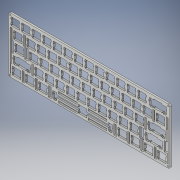
# Autodesk Inventor part: TopPlate
Saved by Autodesk Inventor 2019 (Build 230136000, 136)
## iProperties
Created: 2019-01-24
Part Number: TopPlate
Material: Generic
Document SubType Name: Modeling
Designer: Andrew
Density: 1 g/cm^3
Appearance: Default
Author: Andrew
Autodesk Inventor part; units mm, degrees
(part 1 of 2)
ref_plane "YZ Plane" through (0, 0, 0) normal (1, 0, 0) x (0, 1, 0)
ref_plane "XZ Plane" through (0, 0, 0) normal (0, 1, 0) x (-1, 0, 0)
ref_plane "XY Plane" through (0, 0, 0) normal (0, 0, 1) x (1, 0, 0)
sketch "Sketch1" plane through (0, 0, 0) normal (0, 0, 1) x (1, 0, 0)
  line L0 (290.7004, 97.1993) -> (290.7004, 3)
  arc A0 (287.7004, 0) -> (290.7004, 3) centre (287.7004, 3) ccw
  arc A1 (290.7004, 97.1993) -> (287.7004, 100.1993) centre (287.7004, 97.1993) ccw
  line L1 (126.4424, 18.9995) -> (126.4424, 17.999)
  line L2 (126.4424, 17.999) -> (125.6434, 17.999)
  line L3 (125.6434, 17.999) -> (125.6434, 14.299)
  line L4 (125.6434, 14.299) -> (86.8185, 14.299)
  line L5 (86.8185, 14.299) -> (86.8185, 17.5291)
  line L6 (86.8185, 17.5291) -> (80.0688, 17.5291)
  line L7 (80.0688, 17.5291) -> (80.0688, 14.299)
  line L8 (80.0688, 14.299) -> (79.2433, 14.299)
  line L9 (79.2433, 14.299) -> (79.2433, 11.4989)
  line L10 (79.2433, 11.4989) -> (80.0688, 11.4989)
  line L11 (80.0688, 11.4989) -> (80.0688, 5.2301)
  line L12 (80.0688, 5.2301) -> (81.7924, 5.2301)
  line L13 (81.7924, 5.2301) -> (81.7924, 4.0299)
  line L14 (81.7924, 4.0299) -> (85.093, 4.0299)
  line L15 (85.093, 4.0299) -> (85.093, 5.2301)
  line L16 (85.093, 5.2301) -> (86.8185, 5.2301)
  line L17 (86.8185, 5.2301) -> (86.8185, 9.7005)
  line L18 (86.8185, 9.7005) -> (125.6434, 9.7005)
  line L19 (125.6434, 9.7005) -> (125.6434, 5.9991)
  line L20 (125.6434, 5.9991) -> (126.4424, 5.9991)
  line L21 (126.4424, 5.9991) -> (126.4424, 5)
  line L22 (126.4424, 5) -> (140.4434, 5)
  line L23 (140.4434, 5) -> (140.4434, 5.9991)
  line L24 (140.4434, 5.9991) -> (141.2424, 5.9991)
  line L25 (141.2424, 5.9991) -> (141.2424, 9.7005)
  line L26 (141.2424, 9.7005) -> (180.0694, 9.7005)
  line L27 (180.0694, 9.7005) -> (180.0694, 5.2301)
  line L28 (180.0694, 5.2301) -> (181.7924, 5.2301)
  line L29 (181.7924, 5.2301) -> (181.7924, 4.0299)
  line L30 (181.7924, 4.0299) -> (185.0934, 4.0299)
  line L31 (185.0934, 4.0299) -> (185.0934, 5.2301)
  line L32 (185.0934, 5.2301) -> (186.8184, 5.2301)
  line L33 (186.8184, 5.2301) -> (186.8184, 11.4989)
  line L34 (186.8184, 11.4989) -> (187.6424, 11.4989)
  line L35 (187.6424, 11.4989) -> (187.6424, 14.299)
  line L36 (187.6424, 14.299) -> (186.8184, 14.299)
  line L37 (186.8184, 14.299) -> (186.8184, 17.5291)
  line L38 (186.8184, 17.5291) -> (180.0694, 17.5291)
  line L39 (180.0694, 17.5291) -> (180.0694, 14.299)
  line L40 (180.0694, 14.299) -> (141.2424, 14.299)
  line L41 (141.2424, 14.299) -> (141.2424, 17.999)
  line L42 (141.2424, 17.999) -> (140.4434, 17.999)
  line L43 (140.4434, 17.999) -> (140.4434, 18.9995)
  line L44 (140.4434, 18.9995) -> (126.4424, 18.9995)
  line L45 (7.3813, 18.9995) -> (7.3813, 17.999)
  line L46 (7.3813, 17.999) -> (6.5806, 17.999)
  line L47 (6.5806, 17.999) -> (6.5806, 14.8998)
  line L48 (6.5806, 14.8998) -> (7.3813, 14.8998)
  line L49 (7.3813, 14.8998) -> (7.3813, 9.0997)
  line L50 (7.3813, 9.0997) -> (6.5806, 9.0997)
  line L51 (6.5806, 9.0997) -> (6.5806, 5.9991)
  line L52 (6.5806, 5.9991) -> (7.3813, 5.9991)
  line L53 (7.3813, 5.9991) -> (7.3813, 5)
  line L54 (7.3813, 5) -> (21.3808, 5)
  line L55 (21.3808, 5) -> (21.3808, 5.9991)
  line L56 (21.3808, 5.9991) -> (22.1814, 5.9991)
  line L57 (22.1814, 5.9991) -> (22.1814, 9.0997)
  line L58 (22.1814, 9.0997) -> (21.3808, 9.0997)
  line L59 (21.3808, 9.0997) -> (21.3808, 14.8998)
  line L60 (21.3808, 14.8998) -> (22.1814, 14.8998)
  line L61 (22.1814, 14.8998) -> (22.1814, 17.999)
  line L62 (22.1814, 17.999) -> (21.3808, 17.999)
  line L63 (21.3808, 17.999) -> (21.3808, 18.9995)
  line L64 (21.3808, 18.9995) -> (7.3813, 18.9995)
  line L65 (31.1938, 18.9995) -> (31.1938, 17.999)
  line L66 (31.1938, 17.999) -> (30.3932, 17.999)
  line L67 (30.3932, 17.999) -> (30.3932, 14.8998)
  line L68 (30.3932, 14.8998) -> (31.1938, 14.8998)
  line L69 (31.1938, 14.8998) -> (31.1938, 9.0997)
  line L70 (31.1938, 9.0997) -> (30.3932, 9.0997)
  line L71 (30.3932, 9.0997) -> (30.3932, 5.9991)
  line L72 (30.3932, 5.9991) -> (31.1938, 5.9991)
  line L73 (31.1938, 5.9991) -> (31.1938, 5)
  line L74 (31.1938, 5) -> (45.1932, 5)
  line L75 (45.1932, 5) -> (45.1932, 5.9991)
  line L76 (45.1932, 5.9991) -> (45.9926, 5.9991)
  line L77 (45.9926, 5.9991) -> (45.9926, 9.0997)
  line L78 (45.9926, 9.0997) -> (45.1932, 9.0997)
  line L79 (45.1932, 9.0997) -> (45.1932, 14.8998)
  line L80 (45.1932, 14.8998) -> (45.9926, 14.8998)
  line L81 (45.9926, 14.8998) -> (45.9926, 17.999)
  line L82 (45.9926, 17.999) -> (45.1932, 17.999)
  line L83 (45.1932, 17.999) -> (45.1932, 18.9995)
  line L84 (45.1932, 18.9995) -> (31.1938, 18.9995)
  line L85 (55.0064, 18.9995) -> (55.0064, 17.999)
  line L86 (55.0064, 17.999) -> (54.2056, 17.999)
  line L87 (54.2056, 17.999) -> (54.2056, 14.8998)
  line L88 (54.2056, 14.8998) -> (55.0064, 14.8998)
  line L89 (55.0064, 14.8998) -> (55.0064, 9.0997)
  line L90 (55.0064, 9.0997) -> (54.2056, 9.0997)
  line L91 (54.2056, 9.0997) -> (54.2056, 5.9991)
  line L92 (54.2056, 5.9991) -> (55.0064, 5.9991)
  line L93 (55.0064, 5.9991) -> (55.0064, 5)
  line L94 (55.0064, 5) -> (69.0057, 5)
  line L95 (3, 0) -> (287.7004, 0)
  arc A2 (0, 3) -> (3, 0) centre (3, 3) ccw
  line L96 (69.0057, 5) -> (69.0057, 5.9991)
  line L97 (69.0057, 5.9991) -> (69.8065, 5.9991)
  line L98 (69.8065, 5.9991) -> (69.8065, 9.0997)
  line L99 (69.8065, 9.0997) -> (69.0057, 9.0997)
  line L100 (69.0057, 9.0997) -> (69.0057, 14.8998)
  line L101 (69.0057, 14.8998) -> (69.8065, 14.8998)
  line L102 (69.8065, 14.8998) -> (69.8065, 17.999)
  line L103 (69.8065, 17.999) -> (69.0057, 17.999)
  line L104 (69.0057, 17.999) -> (69.0057, 18.9995)
  line L105 (69.0057, 18.9995) -> (55.0064, 18.9995)
  line L106 (197.8814, 18.9995) -> (197.8814, 17.999)
  line L107 (197.8814, 17.999) -> (197.0804, 17.999)
  line L108 (197.0804, 17.999) -> (197.0804, 14.8998)
  line L109 (197.0804, 14.8998) -> (197.8814, 14.8998)
  line L110 (197.8814, 14.8998) -> (197.8814, 9.0997)
  line L111 (197.8814, 9.0997) -> (197.0804, 9.0997)
  line L112 (197.0804, 9.0997) -> (197.0804, 5.9991)
  line L113 (197.0804, 5.9991) -> (197.8814, 5.9991)
  line L114 (197.8814, 5.9991) -> (197.8814, 5)
  line L115 (197.8814, 5) -> (211.8804, 5)
  line L116 (211.8804, 5) -> (211.8804, 5.9991)
  line L117 (211.8804, 5.9991) -> (212.6814, 5.9991)
  line L118 (212.6814, 5.9991) -> (212.6814, 9.0997)
  line L119 (212.6814, 9.0997) -> (211.8804, 9.0997)
  line L120 (211.8804, 9.0997) -> (211.8804, 14.8998)
  line L121 (211.8804, 14.8998) -> (212.6814, 14.8998)
  line L122 (212.6814, 14.8998) -> (212.6814, 17.999)
  line L123 (212.6814, 17.999) -> (211.8804, 17.999)
  line L124 (211.8804, 17.999) -> (211.8804, 18.9995)
  line L125 (211.8804, 18.9995) -> (197.8814, 18.9995)
  line L126 (221.6934, 18.9995) -> (221.6934, 17.999)
  line L127 (221.6934, 17.999) -> (220.8934, 17.999)
  line L128 (220.8934, 17.999) -> (220.8934, 14.8998)
  line L129 (220.8934, 14.8998) -> (221.6934, 14.8998)
  line L130 (221.6934, 14.8998) -> (221.6934, 9.0997)
  line L131 (221.6934, 9.0997) -> (220.8934, 9.0997)
  line L132 (220.8934, 9.0997) -> (220.8934, 5.9991)
  line L133 (220.8934, 5.9991) -> (221.6934, 5.9991)
  line L134 (221.6934, 5.9991) -> (221.6934, 5)
  line L135 (221.6934, 5) -> (235.6934, 5)
  line L136 (235.6934, 5) -> (235.6934, 5.9991)
  line L137 (235.6934, 5.9991) -> (236.4924, 5.9991)
  line L138 (236.4924, 5.9991) -> (236.4924, 9.0997)
  line L139 (236.4924, 9.0997) -> (235.6934, 9.0997)
  line L140 (235.6934, 9.0997) -> (235.6934, 14.8998)
  line L141 (235.6934, 14.8998) -> (236.4924, 14.8998)
  line L142 (236.4924, 14.8998) -> (236.4924, 17.999)
  line L143 (236.4924, 17.999) -> (235.6934, 17.999)
  line L144 (235.6934, 17.999) -> (235.6934, 18.9995)
  line L145 (235.6934, 18.9995) -> (221.6934, 18.9995)
  line L146 (245.5064, 18.9995) -> (245.5064, 17.999)
  line L147 (245.5064, 17.999) -> (244.7054, 17.999)
  line L148 (244.7054, 17.999) -> (244.7054, 14.8998)
  line L149 (244.7054, 14.8998) -> (245.5064, 14.8998)
  line L150 (245.5064, 14.8998) -> (245.5064, 9.0997)
  line L151 (245.5064, 9.0997) -> (244.7054, 9.0997)
  line L152 (244.7054, 9.0997) -> (244.7054, 5.9991)
  line L153 (244.7054, 5.9991) -> (245.5064, 5.9991)
  line L154 (245.5064, 5.9991) -> (245.5064, 5)
  line L155 (245.5064, 5) -> (259.5054, 5)
  line L156 (259.5054, 5) -> (259.5054, 5.9991)
  line L157 (259.5054, 5.9991) -> (260.3064, 5.9991)
  line L158 (260.3064, 5.9991) -> (260.3064, 9.0997)
  line L159 (260.3064, 9.0997) -> (259.5054, 9.0997)
  line L160 (259.5054, 9.0997) -> (259.5054, 14.8998)
  line L161 (259.5054, 14.8998) -> (260.3064, 14.8998)
  line L162 (260.3064, 14.8998) -> (260.3064, 17.999)
  line L163 (260.3064, 17.999) -> (259.5054, 17.999)
  line L164 (259.5054, 17.999) -> (259.5054, 18.9995)
  line L165 (259.5054, 18.9995) -> (245.5064, 18.9995)
  line L166 (269.3184, 18.9995) -> (269.3184, 17.999)
  line L167 (269.3184, 17.999) -> (268.5184, 17.999)
  line L168 (268.5184, 17.999) -> (268.5184, 14.8998)
  line L169 (268.5184, 14.8998) -> (269.3184, 14.8998)
  line L170 (269.3184, 14.8998) -> (269.3184, 9.0997)
  line L171 (269.3184, 9.0997) -> (268.5184, 9.0997)
  line L172 (268.5184, 9.0997) -> (268.5184, 5.9991)
  line L173 (268.5184, 5.9991) -> (269.3184, 5.9991)
  line L174 (269.3184, 5.9991) -> (269.3184, 5)
  line L175 (269.3184, 5) -> (283.3184, 5)
  line L176 (283.3184, 5) -> (283.3184, 5.9991)
  line L177 (283.3184, 5.9991) -> (284.1174, 5.9991)
  line L178 (284.1174, 5.9991) -> (284.1174, 9.0997)
  line L179 (284.1174, 9.0997) -> (283.3184, 9.0997)
  line L180 (283.3184, 9.0997) -> (283.3184, 14.8998)
  line L181 (283.3184, 14.8998) -> (284.1174, 14.8998)
  line L182 (284.1174, 14.8998) -> (284.1174, 17.999)
  line L183 (284.1174, 17.999) -> (283.3184, 17.999)
  line L184 (283.3184, 17.999) -> (283.3184, 18.9995)
  line L185 (283.3184, 18.9995) -> (269.3184, 18.9995)
  line L186 (16.9063, 38.0493) -> (16.9063, 37.049)
  line L187 (16.9063, 37.049) -> (16.1057, 37.049)
  line L188 (16.1057, 36.5791) -> (8.6312, 36.5791)
  line L189 (8.6312, 36.5791) -> (8.6312, 33.349)
  line L190 (8.6312, 33.349) -> (7.8057, 33.349)
  line L191 (7.8057, 33.349) -> (7.8057, 30.5488)
  line L192 (7.8057, 30.5488) -> (8.6312, 30.5488)
  line L193 (8.6312, 30.5488) -> (8.6312, 24.2787)
  line L194 (8.6312, 24.2787) -> (10.3564, 24.2787)
  line L195 (10.3564, 24.2787) -> (10.3564, 23.0798)
  line L196 (10.3564, 23.0798) -> (13.6555, 23.0798)
  line L197 (13.6555, 23.0798) -> (13.6555, 24.2787)
  line L198 (13.6555, 24.2787) -> (15.3808, 24.2787)
  line L199 (15.3808, 25.049) -> (16.9063, 25.049)
  line L200 (16.9063, 25.049) -> (16.9063, 24.05)
  line L201 (16.9063, 24.05) -> (30.9058, 24.05)
  line L202 (30.9058, 24.05) -> (30.9058, 25.049)
  line L203 (30.9058, 25.049) -> (32.4313, 25.049)
  line L204 (32.4313, 24.2787) -> (34.1566, 24.2787)
  line L205 (34.1566, 24.2787) -> (34.1566, 23.0798)
  line L206 (34.1566, 23.0798) -> (37.4556, 23.0798)
  line L207 (37.4556, 23.0798) -> (37.4556, 24.2787)
  line L208 (37.4556, 24.2787) -> (39.1808, 24.2787)
  line L209 (39.1808, 24.2787) -> (39.1808, 30.5488)
  line L210 (39.1808, 30.5488) -> (40.0063, 30.5488)
  line L211 (40.0063, 30.5488) -> (40.0063, 33.349)
  line L212 (40.0063, 33.349) -> (39.1808, 33.349)
  line L213 (39.1808, 33.349) -> (39.1808, 36.5791)
  line L214 (39.1808, 36.5791) -> (31.7064, 36.5791)
  line L215 (31.7064, 37.049) -> (30.9058, 37.049)
  line L216 (30.9058, 37.049) -> (30.9058, 38.0493)
  line L217 (30.9058, 38.0493) -> (16.9063, 38.0493)
  line L218 (255.0304, 38.0493) -> (255.0304, 37.049)
  line L219 (255.0304, 37.049) -> (254.2304, 37.049)
  line L220 (254.2304, 36.5791) -> (246.7564, 36.5791)
  line L221 (246.7564, 36.5791) -> (246.7564, 33.349)
  line L222 (246.7564, 33.349) -> (245.9304, 33.349)
  line L223 (245.9304, 33.349) -> (245.9304, 30.5488)
  line L224 (245.9304, 30.5488) -> (246.7564, 30.5488)
  line L225 (246.7564, 30.5488) -> (246.7564, 24.2787)
  line L226 (246.7564, 24.2787) -> (248.4814, 24.2787)
  line L227 (248.4814, 24.2787) -> (248.4814, 23.0798)
  line L228 (248.4814, 23.0798) -> (251.7804, 23.0798)
  line L229 (251.7804, 23.0798) -> (251.7804, 24.2787)
  line L230 (251.7804, 24.2787) -> (253.5064, 24.2787)
  line L231 (253.5064, 25.049) -> (255.0304, 25.049)
  line L232 (255.0304, 25.049) -> (255.0304, 24.05)
  line L233 (255.0304, 24.05) -> (269.0304, 24.05)
  line L234 (269.0304, 24.05) -> (269.0304, 25.049)
  line L235 (269.0304, 25.049) -> (270.5564, 25.049)
  line L236 (270.5564, 24.2787) -> (272.2814, 24.2787)
  line L237 (272.2814, 24.2787) -> (272.2814, 23.0798)
  line L238 (272.2814, 23.0798) -> (275.5804, 23.0798)
  line L239 (275.5804, 23.0798) -> (275.5804, 24.2787)
  line L240 (275.5804, 24.2787) -> (277.3054, 24.2787)
  line L241 (277.3054, 24.2787) -> (277.3054, 30.5488)
  line L242 (277.3054, 30.5488) -> (278.1314, 30.5488)
  line L243 (278.1314, 30.5488) -> (278.1314, 33.349)
  line L244 (278.1314, 33.349) -> (277.3054, 33.349)
  line L245 (277.3054, 33.349) -> (277.3054, 36.5791)
  line L246 (277.3054, 36.5791) -> (269.8314, 36.5791)
  line L247 (269.8314, 37.049) -> (269.0304, 37.049)
  line L248 (269.0304, 37.049) -> (269.0304, 38.0493)
  line L249 (269.0304, 38.0493) -> (255.0304, 38.0493)
  line L250 (47.8626, 38.0493) -> (47.8626, 37.049)
  line L251 (47.8626, 37.049) -> (47.0618, 37.049)
  line L252 (47.0618, 37.049) -> (47.0618, 33.9498)
  line L253 (47.0618, 33.9498) -> (47.8626, 33.9498)
  line L254 (47.8626, 33.9498) -> (47.8626, 28.1496)
  line L255 (47.8626, 28.1496) -> (47.0618, 28.1496)
  line L256 (47.0618, 28.1496) -> (47.0618, 25.049)
  line L257 (47.0618, 25.049) -> (47.8626, 25.049)
  line L258 (47.8626, 25.049) -> (47.8626, 24.05)
  line L259 (47.8626, 24.05) -> (61.8619, 24.05)
  line L260 (61.8619, 24.05) -> (61.8619, 25.049)
  line L261 (61.8619, 25.049) -> (62.6627, 25.049)
  line L262 (62.6627, 25.049) -> (62.6627, 28.1496)
  line L263 (62.6627, 28.1496) -> (61.8619, 28.1496)
  line L264 (61.8619, 28.1496) -> (61.8619, 33.9498)
  line L265 (61.8619, 33.9498) -> (62.6627, 33.9498)
  line L266 (62.6627, 33.9498) -> (62.6627, 37.049)
  line L267 (62.6627, 37.049) -> (61.8619, 37.049)
  line L268 (61.8619, 37.049) -> (61.8619, 38.0493)
  line L269 (61.8619, 38.0493) -> (47.8626, 38.0493)
  line L270 (66.9126, 38.0493) -> (66.9126, 37.049)
  line L271 (66.9126, 37.049) -> (66.1118, 37.049)
  line L272 (66.1118, 37.049) -> (66.1118, 33.9498)
  line L273 (66.1118, 33.9498) -> (66.9126, 33.9498)
  line L274 (66.9126, 33.9498) -> (66.9126, 28.1496)
  line L275 (66.9126, 28.1496) -> (66.1118, 28.1496)
  line L276 (66.1118, 28.1496) -> (66.1118, 25.049)
  line L277 (66.1118, 25.049) -> (66.9126, 25.049)
  line L278 (66.9126, 25.049) -> (66.9126, 24.05)
  line L279 (66.9126, 24.05) -> (80.9119, 24.05)
  line L280 (80.9119, 24.05) -> (80.9119, 25.049)
  line L281 (80.9119, 25.049) -> (81.7127, 25.049)
  line L282 (81.7127, 25.049) -> (81.7127, 28.1496)
  line L283 (81.7127, 28.1496) -> (80.9119, 28.1496)
  line L284 (80.9119, 28.1496) -> (80.9119, 33.9498)
  line L285 (80.9119, 33.9498) -> (81.7127, 33.9498)
  line L286 (81.7127, 33.9498) -> (81.7127, 37.049)
  line L287 (81.7127, 37.049) -> (80.9119, 37.049)
  line L288 (80.9119, 37.049) -> (80.9119, 38.0493)
  line L289 (80.9119, 38.0493) -> (66.9126, 38.0493)
  line L290 (85.9626, 38.0493) -> (85.9626, 37.049)
  line L291 (85.9626, 37.049) -> (85.1618, 37.049)
  line L292 (85.1618, 37.049) -> (85.1618, 33.9498)
  line L293 (85.1618, 33.9498) -> (85.9626, 33.9498)
  line L294 (85.9626, 33.9498) -> (85.9626, 28.1496)
  line L295 (85.9626, 28.1496) -> (85.1618, 28.1496)
  line L296 (85.1618, 28.1496) -> (85.1618, 25.049)
  line L297 (85.1618, 25.049) -> (85.9626, 25.049)
  line L298 (85.9626, 25.049) -> (85.9626, 24.05)
  line L299 (85.9626, 24.05) -> (99.9619, 24.05)
  line L300 (99.9619, 24.05) -> (99.9619, 25.049)
  line L301 (99.9619, 25.049) -> (100.7627, 25.049)
  line L302 (100.7627, 25.049) -> (100.7627, 28.1496)
  line L303 (100.7627, 28.1496) -> (99.9619, 28.1496)
  line L304 (99.9619, 28.1496) -> (99.9619, 33.9498)
  line L305 (99.9619, 33.9498) -> (100.7627, 33.9498)
  line L306 (100.7627, 33.9498) -> (100.7627, 37.049)
  line L307 (100.7627, 37.049) -> (99.9619, 37.049)
  line L308 (99.9619, 37.049) -> (99.9619, 38.0493)
  line L309 (99.9619, 38.0493) -> (85.9626, 38.0493)
  line L310 (105.0124, 38.0493) -> (105.0124, 37.049)
  line L311 (105.0124, 37.049) -> (104.2114, 37.049)
  line L312 (104.2114, 37.049) -> (104.2114, 33.9498)
  line L313 (104.2114, 33.9498) -> (105.0124, 33.9498)
  line L314 (105.0124, 33.9498) -> (105.0124, 28.1496)
  line L315 (105.0124, 28.1496) -> (104.2114, 28.1496)
  line L316 (104.2114, 28.1496) -> (104.2114, 25.049)
  line L317 (104.2114, 25.049) -> (105.0124, 25.049)
  line L318 (105.0124, 25.049) -> (105.0124, 24.05)
  line L319 (105.0124, 24.05) -> (119.0124, 24.05)
  line L320 (119.0124, 24.05) -> (119.0124, 25.049)
  line L321 (119.0124, 25.049) -> (119.8124, 25.049)
  line L322 (119.8124, 25.049) -> (119.8124, 28.1496)
  line L323 (119.8124, 28.1496) -> (119.0124, 28.1496)
  line L324 (119.0124, 28.1496) -> (119.0124, 33.9498)
  line L325 (119.0124, 33.9498) -> (119.8124, 33.9498)
  line L326 (119.8124, 33.9498) -> (119.8124, 37.049)
  line L327 (119.8124, 37.049) -> (119.0124, 37.049)
  line L328 (119.0124, 37.049) -> (119.0124, 38.0493)
  line L329 (119.0124, 38.0493) -> (105.0124, 38.0493)
  line L330 (124.0624, 38.0493) -> (124.0624, 37.049)
  line L331 (124.0624, 37.049) -> (123.2614, 37.049)
  line L332 (123.2614, 37.049) -> (123.2614, 33.9498)
  line L333 (123.2614, 33.9498) -> (124.0624, 33.9498)
  line L334 (124.0624, 33.9498) -> (124.0624, 28.1496)
  line L335 (124.0624, 28.1496) -> (123.2614, 28.1496)
  line L336 (123.2614, 28.1496) -> (123.2614, 25.049)
  line L337 (123.2614, 25.049) -> (124.0624, 25.049)
  line L338 (124.0624, 25.049) -> (124.0624, 24.05)
  line L339 (124.0624, 24.05) -> (138.0624, 24.05)
  line L340 (138.0624, 24.05) -> (138.0624, 25.049)
  line L341 (138.0624, 25.049) -> (138.8624, 25.049)
  line L342 (138.8624, 25.049) -> (138.8624, 28.1496)
  line L343 (138.8624, 28.1496) -> (138.0624, 28.1496)
  line L344 (138.0624, 28.1496) -> (138.0624, 33.9498)
  line L345 (138.0624, 33.9498) -> (138.8624, 33.9498)
  line L346 (138.8624, 33.9498) -> (138.8624, 37.049)
  line L347 (138.8624, 37.049) -> (138.0624, 37.049)
  line L348 (138.0624, 37.049) -> (138.0624, 38.0493)
  line L349 (138.0624, 38.0493) -> (124.0624, 38.0493)
  line L350 (143.1124, 38.0493) -> (143.1124, 37.049)
  line L351 (143.1124, 37.049) -> (142.3114, 37.049)
  line L352 (142.3114, 37.049) -> (142.3114, 33.9498)
  line L353 (142.3114, 33.9498) -> (143.1124, 33.9498)
  line L354 (143.1124, 33.9498) -> (143.1124, 28.1496)
  line L355 (143.1124, 28.1496) -> (142.3114, 28.1496)
  line L356 (142.3114, 28.1496) -> (142.3114, 25.049)
  line L357 (142.3114, 25.049) -> (143.1124, 25.049)
  line L358 (143.1124, 25.049) -> (143.1124, 24.05)
  line L359 (143.1124, 24.05) -> (157.1124, 24.05)
  line L360 (157.1124, 24.05) -> (157.1124, 25.049)
  line L361 (157.1124, 25.049) -> (157.9124, 25.049)
  line L362 (157.9124, 25.049) -> (157.9124, 28.1496)
  line L363 (157.9124, 28.1496) -> (157.1124, 28.1496)
  line L364 (157.1124, 28.1496) -> (157.1124, 33.9498)
  line L365 (157.1124, 33.9498) -> (157.9124, 33.9498)
  line L366 (157.9124, 33.9498) -> (157.9124, 37.049)
  line L367 (157.9124, 37.049) -> (157.1124, 37.049)
  line L368 (157.1124, 37.049) -> (157.1124, 38.0493)
  line L369 (157.1124, 38.0493) -> (143.1124, 38.0493)
  line L370 (162.1624, 38.0493) -> (162.1624, 37.049)
  line L371 (162.1624, 37.049) -> (161.3614, 37.049)
  line L372 (161.3614, 37.049) -> (161.3614, 33.9498)
  line L373 (161.3614, 33.9498) -> (162.1624, 33.9498)
  line L374 (162.1624, 33.9498) -> (162.1624, 28.1496)
  line L375 (162.1624, 28.1496) -> (161.3614, 28.1496)
  line L376 (161.3614, 28.1496) -> (161.3614, 25.049)
  line L377 (161.3614, 25.049) -> (162.1624, 25.049)
  line L378 (162.1624, 25.049) -> (162.1624, 24.05)
  line L379 (162.1624, 24.05) -> (176.1624, 24.05)
  line L380 (176.1624, 24.05) -> (176.1624, 25.049)
  line L381 (176.1624, 25.049) -> (176.9624, 25.049)
  line L382 (176.9624, 25.049) -> (176.9624, 28.1496)
  line L383 (176.9624, 28.1496) -> (176.1624, 28.1496)
  line L384 (176.1624, 28.1496) -> (176.1624, 33.9498)
  line L385 (176.1624, 33.9498) -> (176.9624, 33.9498)
  line L386 (176.9624, 33.9498) -> (176.9624, 37.049)
  line L387 (176.9624, 37.049) -> (176.1624, 37.049)
  line L388 (176.1624, 37.049) -> (176.1624, 38.0493)
  line L389 (176.1624, 38.0493) -> (162.1624, 38.0493)
  line L390 (181.2124, 38.0493) -> (181.2124, 37.049)
  line L391 (181.2124, 37.049) -> (180.4114, 37.049)
  line L392 (180.4114, 37.049) -> (180.4114, 33.9498)
  line L393 (180.4114, 33.9498) -> (181.2124, 33.9498)
  line L394 (181.2124, 33.9498) -> (181.2124, 28.1496)
  line L395 (181.2124, 28.1496) -> (180.4114, 28.1496)
  line L396 (180.4114, 28.1496) -> (180.4114, 25.049)
  line L397 (180.4114, 25.049) -> (181.2124, 25.049)
  line L398 (181.2124, 25.049) -> (181.2124, 24.05)
  line L399 (181.2124, 24.05) -> (195.2124, 24.05)
  line L400 (195.2124, 24.05) -> (195.2124, 25.049)
  line L401 (195.2124, 25.049) -> (196.0124, 25.049)
  line L402 (196.0124, 25.049) -> (196.0124, 28.1496)
  line L403 (196.0124, 28.1496) -> (195.2124, 28.1496)
  line L404 (195.2124, 28.1496) -> (195.2124, 33.9498)
  line L405 (195.2124, 33.9498) -> (196.0124, 33.9498)
  line L406 (196.0124, 33.9498) -> (196.0124, 37.049)
  line L407 (196.0124, 37.049) -> (195.2124, 37.049)
  line L408 (195.2124, 37.049) -> (195.2124, 38.0493)
  line L409 (195.2124, 38.0493) -> (181.2124, 38.0493)
  line L410 (200.2624, 38.0493) -> (200.2624, 37.049)
  line L411 (200.2624, 37.049) -> (199.4614, 37.049)
  line L412 (199.4614, 37.049) -> (199.4614, 33.9498)
  line L413 (199.4614, 33.9498) -> (200.2624, 33.9498)
  line L414 (200.2624, 33.9498) -> (200.2624, 28.1496)
  line L415 (200.2624, 28.1496) -> (199.4614, 28.1496)
  line L416 (199.4614, 28.1496) -> (199.4614, 25.049)
  line L417 (199.4614, 25.049) -> (200.2624, 25.049)
  line L418 (200.2624, 25.049) -> (200.2624, 24.05)
  line L419 (200.2624, 24.05) -> (214.2624, 24.05)
  line L420 (214.2624, 24.05) -> (214.2624, 25.049)
  line L421 (214.2624, 25.049) -> (215.0624, 25.049)
  line L422 (215.0624, 25.049) -> (215.0624, 28.1496)
  line L423 (215.0624, 28.1496) -> (214.2624, 28.1496)
  line L424 (214.2624, 28.1496) -> (214.2624, 33.9498)
  line L425 (214.2624, 33.9498) -> (215.0624, 33.9498)
  line L426 (215.0624, 33.9498) -> (215.0624, 37.049)
  line L427 (215.0624, 37.049) -> (214.2624, 37.049)
  line L428 (214.2624, 37.049) -> (214.2624, 38.0493)
  line L429 (214.2624, 38.0493) -> (200.2624, 38.0493)
  line L430 (219.3124, 38.0493) -> (219.3124, 37.049)
  line L431 (219.3124, 37.049) -> (218.5114, 37.049)
  line L432 (218.5114, 37.049) -> (218.5114, 33.9498)
  line L433 (218.5114, 33.9498) -> (219.3124, 33.9498)
  line L434 (219.3124, 33.9498) -> (219.3124, 28.1496)
  line L435 (219.3124, 28.1496) -> (218.5114, 28.1496)
  line L436 (218.5114, 28.1496) -> (218.5114, 25.049)
  line L437 (218.5114, 25.049) -> (219.3124, 25.049)
  line L438 (219.3124, 25.049) -> (219.3124, 24.05)
  line L439 (219.3124, 24.05) -> (233.3124, 24.05)
  line L440 (233.3124, 24.05) -> (233.3124, 25.049)
  line L441 (233.3124, 25.049) -> (234.1124, 25.049)
  line L442 (234.1124, 25.049) -> (234.1124, 28.1496)
  line L443 (234.1124, 28.1496) -> (233.3124, 28.1496)
  line L444 (233.3124, 28.1496) -> (233.3124, 33.9498)
  line L445 (233.3124, 33.9498) -> (234.1124, 33.9498)
  line L446 (234.1124, 33.9498) -> (234.1124, 37.049)
  line L447 (234.1124, 37.049) -> (233.3124, 37.049)
  line L448 (233.3124, 37.049) -> (233.3124, 38.0493)
  line L449 (233.3124, 38.0493) -> (219.3124, 38.0493)
  line L450 (259.7934, 57.0993) -> (259.7934, 56.0992)
  line L451 (259.7934, 56.0992) -> (258.9914, 56.0992)
  line L452 (258.9914, 56.0992) -> (258.9914, 55.6293)
  line L453 (258.9914, 55.6293) -> (251.5184, 55.6293)
  line L454 (251.5184, 55.6293) -> (251.5184, 52.3989)
  line L455 (251.5184, 52.3989) -> (250.6934, 52.3989)
  line L456 (250.6934, 52.3989) -> (250.6934, 49.5989)
  line L457 (250.6934, 49.5989) -> (251.5184, 49.5989)
  line L458 (251.5184, 49.5989) -> (251.5184, 43.33)
  line L459 (251.5184, 43.33) -> (253.2424, 43.33)
  line L460 (253.2424, 43.33) -> (253.2424, 42.1299)
  line L461 (253.2424, 42.1299) -> (256.5414, 42.1299)
  line L462 (256.5414, 42.1299) -> (256.5414, 43.33)
  line L463 (256.5414, 43.33) -> (258.2684, 43.33)
  line L464 (258.2684, 43.33) -> (258.2684, 44.0991)
  line L465 (258.2684, 44.0991) -> (259.7934, 44.0991)
  line L466 (259.7934, 44.0991) -> (259.7934, 43.1)
  line L467 (259.7934, 43.1) -> (273.7934, 43.1)
  line L468 (273.7934, 43.1) -> (273.7934, 44.0991)
  line L469 (273.7934, 44.0991) -> (275.3194, 44.0991)
  line L470 (275.3194, 44.0991) -> (275.3194, 43.33)
  line L471 (275.3194, 43.33) -> (277.0424, 43.33)
  line L472 (277.0424, 43.33) -> (277.0424, 42.1299)
  line L473 (277.0424, 42.1299) -> (280.3434, 42.1299)
  line L474 (280.3434, 42.1299) -> (280.3434, 43.33)
  line L475 (280.3434, 43.33) -> (282.0684, 43.33)
  line L476 (282.0684, 43.33) -> (282.0684, 49.5989)
  line L477 (282.0684, 49.5989) -> (282.8924, 49.5989)
  line L478 (282.8924, 49.5989) -> (282.8924, 52.3989)
  line L479 (282.8924, 52.3989) -> (282.0684, 52.3989)
  line L480 (282.0684, 52.3989) -> (282.0684, 55.6293)
  line L481 (282.0684, 55.6293) -> (274.5924, 55.6293)
  line L482 (274.5924, 55.6293) -> (274.5924, 56.0992)
  line L483 (274.5924, 56.0992) -> (273.7934, 56.0992)
  line L484 (273.7934, 56.0992) -> (273.7934, 57.0993)
  line L485 (273.7934, 57.0993) -> (259.7934, 57.0993)
  line L486 (12.1438, 57.0993) -> (12.1438, 56.0992)
  line L487 (12.1438, 56.0992) -> (11.3431, 56.0992)
  line L488 (11.3431, 56.0992) -> (11.3431, 52.9997)
  line L489 (11.3431, 52.9997) -> (12.1438, 52.9997)
  line L490 (12.1438, 52.9997) -> (12.1438, 47.1996)
  line L491 (12.1438, 47.1996) -> (11.3431, 47.1996)
  line L492 (11.3431, 47.1996) -> (11.3431, 44.0991)
  line L493 (11.3431, 44.0991) -> (12.1438, 44.0991)
  line L494 (12.1438, 44.0991) -> (12.1438, 43.1)
  line L495 (12.1438, 43.1) -> (26.1433, 43.1)
  line L496 (26.1433, 43.1) -> (26.1433, 44.0991)
  line L497 (26.1433, 44.0991) -> (26.9426, 44.0991)
  line L498 (26.9426, 44.0991) -> (26.9426, 47.1996)
  line L499 (26.9426, 47.1996) -> (26.1433, 47.1996)
  line L500 (26.1433, 47.1996) -> (26.1433, 52.9997)
  line L501 (26.1433, 52.9997) -> (26.9426, 52.9997)
  line L502 (26.9426, 52.9997) -> (26.9426, 56.0992)
  line L503 (26.9426, 56.0992) -> (26.1433, 56.0992)
  line L504 (26.1433, 56.0992) -> (26.1433, 57.0993)
  line L505 (26.1433, 57.0993) -> (12.1438, 57.0993)
  line L506 (38.3376, 57.0993) -> (38.3376, 56.0992)
  line L507 (38.3376, 56.0992) -> (37.5369, 56.0992)
  line L508 (37.5369, 56.0992) -> (37.5369, 52.9997)
  line L509 (37.5369, 52.9997) -> (38.3376, 52.9997)
  line L510 (38.3376, 52.9997) -> (38.3376, 47.1996)
  line L511 (38.3376, 47.1996) -> (37.5369, 47.1996)
  line L512 (37.5369, 47.1996) -> (37.5369, 44.0991)
  line L513 (37.5369, 44.0991) -> (38.3376, 44.0991)
  line L514 (38.3376, 44.0991) -> (38.3376, 43.1)
  line L515 (38.3376, 43.1) -> (52.3369, 43.1)
  line L516 (52.3369, 43.1) -> (52.3369, 44.0991)
  line L517 (52.3369, 44.0991) -> (53.1377, 44.0991)
  line L518 (53.1377, 44.0991) -> (53.1377, 47.1996)
  line L519 (53.1377, 47.1996) -> (52.3369, 47.1996)
  line L520 (52.3369, 47.1996) -> (52.3369, 52.9997)
  line L521 (52.3369, 52.9997) -> (53.1377, 52.9997)
  line L522 (53.1377, 52.9997) -> (53.1377, 56.0992)
  line L523 (53.1377, 56.0992) -> (52.3369, 56.0992)
  line L524 (52.3369, 56.0992) -> (52.3369, 57.0993)
  line L525 (52.3369, 57.0993) -> (38.3376, 57.0993)
  line L526 (57.3876, 57.0993) -> (57.3876, 56.0992)
  line L527 (57.3876, 56.0992) -> (56.5868, 56.0992)
  line L528 (56.5868, 56.0992) -> (56.5868, 52.9997)
  line L529 (56.5868, 52.9997) -> (57.3876, 52.9997)
  line L530 (57.3876, 52.9997) -> (57.3876, 47.1996)
  line L531 (57.3876, 47.1996) -> (56.5868, 47.1996)
  line L532 (56.5868, 47.1996) -> (56.5868, 44.0991)
  line L533 (56.5868, 44.0991) -> (57.3876, 44.0991)
  line L534 (57.3876, 44.0991) -> (57.3876, 43.1)
  line L535 (57.3876, 43.1) -> (71.3869, 43.1)
  line L536 (71.3869, 43.1) -> (71.3869, 44.0991)
  line L537 (71.3869, 44.0991) -> (72.1877, 44.0991)
  line L538 (72.1877, 44.0991) -> (72.1877, 47.1996)
  line L539 (72.1877, 47.1996) -> (71.3869, 47.1996)
  line L540 (71.3869, 47.1996) -> (71.3869, 52.9997)
  line L541 (71.3869, 52.9997) -> (72.1877, 52.9997)
  line L542 (72.1877, 52.9997) -> (72.1877, 56.0992)
  line L543 (72.1877, 56.0992) -> (71.3869, 56.0992)
  line L544 (71.3869, 56.0992) -> (71.3869, 57.0993)
  line L545 (71.3869, 57.0993) -> (57.3876, 57.0993)
  line L546 (76.4376, 57.0993) -> (76.4376, 56.0992)
  line L547 (76.4376, 56.0992) -> (75.6368, 56.0992)
  line L548 (75.6368, 56.0992) -> (75.6368, 52.9997)
  line L549 (75.6368, 52.9997) -> (76.4376, 52.9997)
  line L550 (76.4376, 52.9997) -> (76.4376, 47.1996)
  line L551 (76.4376, 47.1996) -> (75.6368, 47.1996)
  line L552 (75.6368, 47.1996) -> (75.6368, 44.0991)
  line L553 (75.6368, 44.0991) -> (76.4376, 44.0991)
  line L554 (76.4376, 44.0991) -> (76.4376, 43.1)
  line L555 (76.4376, 43.1) -> (90.4369, 43.1)
  line L556 (90.4369, 43.1) -> (90.4369, 44.0991)
  line L557 (90.4369, 44.0991) -> (91.2377, 44.0991)
  line L558 (91.2377, 44.0991) -> (91.2377, 47.1996)
  line L559 (91.2377, 47.1996) -> (90.4369, 47.1996)
  line L560 (90.4369, 47.1996) -> (90.4369, 52.9997)
  line L561 (90.4369, 52.9997) -> (91.2377, 52.9997)
  line L562 (91.2377, 52.9997) -> (91.2377, 56.0992)
  line L563 (91.2377, 56.0992) -> (90.4369, 56.0992)
  line L564 (90.4369, 56.0992) -> (90.4369, 57.0993)
  line L565 (90.4369, 57.0993) -> (76.4376, 57.0993)
  line L566 (95.4876, 57.0993) -> (95.4876, 56.0992)
  line L567 (95.4876, 56.0992) -> (94.6868, 56.0992)
  line L568 (94.6868, 56.0992) -> (94.6868, 52.9997)
  line L569 (94.6868, 52.9997) -> (95.4876, 52.9997)
  line L570 (95.4876, 52.9997) -> (95.4876, 47.1996)
  line L571 (95.4876, 47.1996) -> (94.6868, 47.1996)
  line L572 (94.6868, 47.1996) -> (94.6868, 44.0991)
  line L573 (94.6868, 44.0991) -> (95.4876, 44.0991)
  line L574 (95.4876, 44.0991) -> (95.4876, 43.1)
  line L575 (95.4876, 43.1) -> (109.4874, 43.1)
  line L576 (109.4874, 43.1) -> (109.4874, 44.0991)
  line L577 (109.4874, 44.0991) -> (110.2874, 44.0991)
  line L578 (110.2874, 44.0991) -> (110.2874, 47.1996)
  line L579 (110.2874, 47.1996) -> (109.4874, 47.1996)
  line L580 (109.4874, 47.1996) -> (109.4874, 52.9997)
  line L581 (109.4874, 52.9997) -> (110.2874, 52.9997)
  line L582 (110.2874, 52.9997) -> (110.2874, 56.0992)
  line L583 (110.2874, 56.0992) -> (109.4874, 56.0992)
  line L584 (109.4874, 56.0992) -> (109.4874, 57.0993)
  line L585 (109.4874, 57.0993) -> (95.4876, 57.0993)
  line L586 (114.5374, 57.0993) -> (114.5374, 56.0992)
  line L587 (114.5374, 56.0992) -> (113.7364, 56.0992)
  line L588 (113.7364, 56.0992) -> (113.7364, 52.9997)
  line L589 (113.7364, 52.9997) -> (114.5374, 52.9997)
  line L590 (114.5374, 52.9997) -> (114.5374, 47.1996)
  line L591 (114.5374, 47.1996) -> (113.7364, 47.1996)
  line L592 (113.7364, 47.1996) -> (113.7364, 44.0991)
  line L593 (113.7364, 44.0991) -> (114.5374, 44.0991)
  line L594 (114.5374, 44.0991) -> (114.5374, 43.1)
  line L595 (114.5374, 43.1) -> (128.5374, 43.1)
  line L596 (128.5374, 43.1) -> (128.5374, 44.0991)
  line L597 (128.5374, 44.0991) -> (129.3374, 44.0991)
  line L598 (129.3374, 44.0991) -> (129.3374, 47.1996)
  line L599 (129.3374, 47.1996) -> (128.5374, 47.1996)
  line L600 (128.5374, 47.1996) -> (128.5374, 52.9997)
  line L601 (128.5374, 52.9997) -> (129.3374, 52.9997)
  line L602 (129.3374, 52.9997) -> (129.3374, 56.0992)
  line L603 (129.3374, 56.0992) -> (128.5374, 56.0992)
  line L604 (128.5374, 56.0992) -> (128.5374, 57.0993)
  line L605 (128.5374, 57.0993) -> (114.5374, 57.0993)
  line L606 (133.5874, 57.0993) -> (133.5874, 56.0992)
  line L607 (133.5874, 56.0992) -> (132.7864, 56.0992)
  line L608 (132.7864, 56.0992) -> (132.7864, 52.9997)
  line L609 (132.7864, 52.9997) -> (133.5874, 52.9997)
  line L610 (133.5874, 52.9997) -> (133.5874, 47.1996)
  line L611 (133.5874, 47.1996) -> (132.7864, 47.1996)
  line L612 (132.7864, 47.1996) -> (132.7864, 44.0991)
  line L613 (132.7864, 44.0991) -> (133.5874, 44.0991)
  line L614 (133.5874, 44.0991) -> (133.5874, 43.1)
  line L615 (133.5874, 43.1) -> (147.5874, 43.1)
  line L616 (147.5874, 43.1) -> (147.5874, 44.0991)
  line L617 (147.5874, 44.0991) -> (148.3874, 44.0991)
  line L618 (148.3874, 44.0991) -> (148.3874, 47.1996)
  line L619 (148.3874, 47.1996) -> (147.5874, 47.1996)
  line L620 (147.5874, 47.1996) -> (147.5874, 52.9997)
  line L621 (147.5874, 52.9997) -> (148.3874, 52.9997)
  line L622 (148.3874, 52.9997) -> (148.3874, 56.0992)
  line L623 (148.3874, 56.0992) -> (147.5874, 56.0992)
  line L624 (147.5874, 56.0992) -> (147.5874, 57.0993)
  line L625 (147.5874, 57.0993) -> (133.5874, 57.0993)
  line L626 (152.6374, 57.0993) -> (152.6374, 56.0992)
  line L627 (152.6374, 56.0992) -> (151.8364, 56.0992)
  line L628 (151.8364, 56.0992) -> (151.8364, 52.9997)
  line L629 (151.8364, 52.9997) -> (152.6374, 52.9997)
  line L630 (152.6374, 52.9997) -> (152.6374, 47.1996)
  line L631 (152.6374, 47.1996) -> (151.8364, 47.1996)
  line L632 (151.8364, 47.1996) -> (151.8364, 44.0991)
  line L633 (151.8364, 44.0991) -> (152.6374, 44.0991)
  line L634 (152.6374, 44.0991) -> (152.6374, 43.1)
  line L635 (152.6374, 43.1) -> (166.6374, 43.1)
  line L636 (166.6374, 43.1) -> (166.6374, 44.0991)
  line L637 (166.6374, 44.0991) -> (167.4374, 44.0991)
  line L638 (167.4374, 44.0991) -> (167.4374, 47.1996)
  line L639 (167.4374, 47.1996) -> (166.6374, 47.1996)
  line L640 (166.6374, 47.1996) -> (166.6374, 52.9997)
  line L641 (166.6374, 52.9997) -> (167.4374, 52.9997)
  line L642 (167.4374, 52.9997) -> (167.4374, 56.0992)
  line L643 (167.4374, 56.0992) -> (166.6374, 56.0992)
  line L644 (166.6374, 56.0992) -> (166.6374, 57.0993)
  line L645 (166.6374, 57.0993) -> (152.6374, 57.0993)
  line L646 (171.6874, 57.0993) -> (171.6874, 56.0992)
  line L647 (171.6874, 56.0992) -> (170.8864, 56.0992)
  line L648 (170.8864, 56.0992) -> (170.8864, 52.9997)
  line L649 (170.8864, 52.9997) -> (171.6874, 52.9997)
  line L650 (171.6874, 52.9997) -> (171.6874, 47.1996)
  line L651 (171.6874, 47.1996) -> (170.8864, 47.1996)
  line L652 (170.8864, 47.1996) -> (170.8864, 44.0991)
  line L653 (170.8864, 44.0991) -> (171.6874, 44.0991)
  line L654 (171.6874, 44.0991) -> (171.6874, 43.1)
  line L655 (171.6874, 43.1) -> (185.6874, 43.1)
  line L656 (185.6874, 43.1) -> (185.6874, 44.0991)
  line L657 (185.6874, 44.0991) -> (186.4874, 44.0991)
  line L658 (186.4874, 44.0991) -> (186.4874, 47.1996)
  line L659 (186.4874, 47.1996) -> (185.6874, 47.1996)
  line L660 (185.6874, 47.1996) -> (185.6874, 52.9997)
  line L661 (185.6874, 52.9997) -> (186.4874, 52.9997)
  line L662 (186.4874, 52.9997) -> (186.4874, 56.0992)
  line L663 (186.4874, 56.0992) -> (185.6874, 56.0992)
  line L664 (185.6874, 56.0992) -> (185.6874, 57.0993)
  line L665 (185.6874, 57.0993) -> (171.6874, 57.0993)
  line L666 (190.7374, 57.0993) -> (190.7374, 56.0992)
  line L667 (190.7374, 56.0992) -> (189.9364, 56.0992)
  line L668 (189.9364, 56.0992) -> (189.9364, 52.9997)
  line L669 (189.9364, 52.9997) -> (190.7374, 52.9997)
  line L670 (190.7374, 52.9997) -> (190.7374, 47.1996)
  line L671 (190.7374, 47.1996) -> (189.9364, 47.1996)
  line L672 (189.9364, 47.1996) -> (189.9364, 44.0991)
  line L673 (189.9364, 44.0991) -> (190.7374, 44.0991)
  line L674 (190.7374, 44.0991) -> (190.7374, 43.1)
  line L675 (190.7374, 43.1) -> (204.7374, 43.1)
  line L676 (204.7374, 43.1) -> (204.7374, 44.0991)
  line L677 (204.7374, 44.0991) -> (205.5374, 44.0991)
  line L678 (205.5374, 44.0991) -> (205.5374, 47.1996)
  line L679 (205.5374, 47.1996) -> (204.7374, 47.1996)
  line L680 (204.7374, 47.1996) -> (204.7374, 52.9997)
  line L681 (204.7374, 52.9997) -> (205.5374, 52.9997)
  line L682 (205.5374, 52.9997) -> (205.5374, 56.0992)
  line L683 (205.5374, 56.0992) -> (204.7374, 56.0992)
  line L684 (204.7374, 56.0992) -> (204.7374, 57.0993)
  line L685 (204.7374, 57.0993) -> (190.7374, 57.0993)
  line L686 (209.7874, 57.0993) -> (209.7874, 56.0992)
  line L687 (209.7874, 56.0992) -> (208.9864, 56.0992)
  line L688 (208.9864, 56.0992) -> (208.9864, 52.9997)
  line L689 (208.9864, 52.9997) -> (209.7874, 52.9997)
  line L690 (209.7874, 52.9997) -> (209.7874, 47.1996)
  line L691 (209.7874, 47.1996) -> (208.9864, 47.1996)
  line L692 (208.9864, 47.1996) -> (208.9864, 44.0991)
  line L693 (208.9864, 44.0991) -> (209.7874, 44.0991)
  line L694 (209.7874, 44.0991) -> (209.7874, 43.1)
  line L695 (209.7874, 43.1) -> (223.7874, 43.1)
  line L696 (223.7874, 43.1) -> (223.7874, 44.0991)
  line L697 (223.7874, 44.0991) -> (224.5874, 44.0991)
  line L698 (224.5874, 44.0991) -> (224.5874, 47.1996)
  line L699 (224.5874, 47.1996) -> (223.7874, 47.1996)
  line L700 (223.7874, 47.1996) -> (223.7874, 52.9997)
  line L701 (223.7874, 52.9997) -> (224.5874, 52.9997)
  line L702 (224.5874, 52.9997) -> (224.5874, 56.0992)
  line L703 (224.5874, 56.0992) -> (223.7874, 56.0992)
  line L704 (223.7874, 56.0992) -> (223.7874, 57.0993)
  line L705 (223.7874, 57.0993) -> (209.7874, 57.0993)
  line L706 (228.8374, 57.0993) -> (228.8374, 56.0992)
  line L707 (228.8374, 56.0992) -> (228.0364, 56.0992)
  line L708 (228.0364, 56.0992) -> (228.0364, 52.9997)
  line L709 (228.0364, 52.9997) -> (228.8374, 52.9997)
  line L710 (228.8374, 52.9997) -> (228.8374, 47.1996)
  line L711 (228.8374, 47.1996) -> (228.0364, 47.1996)
  line L712 (228.0364, 47.1996) -> (228.0364, 44.0991)
  line L713 (228.0364, 44.0991) -> (228.8374, 44.0991)
  line L714 (228.8374, 44.0991) -> (228.8374, 43.1)
  line L715 (228.8374, 43.1) -> (242.8374, 43.1)
  line L716 (242.8374, 43.1) -> (242.8374, 44.0991)
  line L717 (242.8374, 44.0991) -> (243.6374, 44.0991)
  line L718 (243.6374, 44.0991) -> (243.6374, 47.1996)
  line L719 (243.6374, 47.1996) -> (242.8374, 47.1996)
  line L720 (242.8374, 47.1996) -> (242.8374, 52.9997)
  line L721 (242.8374, 52.9997) -> (243.6374, 52.9997)
  line L722 (243.6374, 52.9997) -> (243.6374, 56.0992)
  line L723 (243.6374, 56.0992) -> (242.8374, 56.0992)
  line L724 (242.8374, 56.0992) -> (242.8374, 57.0993)
  line L725 (242.8374, 57.0993) -> (228.8374, 57.0993)
  line L726 (9.7625, 76.1493) -> (9.7625, 75.1492)
  line L727 (9.7625, 75.1492) -> (8.9619, 75.1492)
  line L728 (8.9619, 75.1492) -> (8.9619, 72.0497)
  line L729 (8.9619, 72.0497) -> (9.7625, 72.0497)
  line L730 (9.7625, 72.0497) -> (9.7625, 66.2496)
  line L731 (9.7625, 66.2496) -> (8.9619, 66.2496)
  line L732 (8.9619, 66.2496) -> (8.9619, 63.1491)
  line L733 (8.9619, 63.1491) -> (9.7625, 63.1491)
  line L734 (9.7625, 63.1491) -> (9.7625, 62.15)
  line L735 (9.7625, 62.15) -> (23.7621, 62.15)
  line L736 (23.7621, 62.15) -> (23.7621, 63.1491)
  line L737 (23.7621, 63.1491) -> (24.5627, 63.1491)
  line L738 (24.5627, 63.1491) -> (24.5627, 66.2496)
  line L739 (24.5627, 66.2496) -> (23.7621, 66.2496)
  line L740 (23.7621, 66.2496) -> (23.7621, 72.0497)
  line L741 (23.7621, 72.0497) -> (24.5627, 72.0497)
  line L742 (24.5627, 72.0497) -> (24.5627, 75.1492)
  line L743 (24.5627, 75.1492) -> (23.7621, 75.1492)
  line L744 (23.7621, 75.1492) -> (23.7621, 76.1493)
  line L745 (23.7621, 76.1493) -> (9.7625, 76.1493)
  line L746 (33.5751, 76.1493) -> (33.5751, 75.1492)
  line L747 (33.5751, 75.1492) -> (32.7758, 75.1492)
  line L748 (32.7758, 75.1492) -> (32.7758, 72.0497)
  line L749 (32.7758, 72.0497) -> (33.5751, 72.0497)
  line L750 (33.5751, 72.0497) -> (33.5751, 66.2496)
  line L751 (33.5751, 66.2496) -> (32.7758, 66.2496)
  line L752 (32.7758, 66.2496) -> (32.7758, 63.1491)
  line L753 (32.7758, 63.1491) -> (33.5751, 63.1491)
  line L754 (33.5751, 63.1491) -> (33.5751, 62.15)
  line L755 (33.5751, 62.15) -> (47.5744, 62.15)
  line L756 (47.5744, 62.15) -> (47.5744, 63.1491)
  line L757 (47.5744, 63.1491) -> (48.3752, 63.1491)
  line L758 (48.3752, 63.1491) -> (48.3752, 66.2496)
  line L759 (48.3752, 66.2496) -> (47.5744, 66.2496)
  line L760 (47.5744, 66.2496) -> (47.5744, 72.0497)
  line L761 (47.5744, 72.0497) -> (48.3752, 72.0497)
  line L762 (48.3752, 72.0497) -> (48.3752, 75.1492)
  line L763 (48.3752, 75.1492) -> (47.5744, 75.1492)
  line L764 (47.5744, 75.1492) -> (47.5744, 76.1493)
  line L765 (47.5744, 76.1493) -> (33.5751, 76.1493)
  line L766 (52.6251, 76.1493) -> (52.6251, 75.1492)
  line L767 (52.6251, 75.1492) -> (51.8257, 75.1492)
  line L768 (51.8257, 75.1492) -> (51.8257, 72.0497)
  line L769 (51.8257, 72.0497) -> (52.6251, 72.0497)
  line L770 (52.6251, 72.0497) -> (52.6251, 66.2496)
  line L771 (52.6251, 66.2496) -> (51.8257, 66.2496)
  line L772 (51.8257, 66.2496) -> (51.8257, 63.1491)
  line L773 (51.8257, 63.1491) -> (52.6251, 63.1491)
  line L774 (52.6251, 63.1491) -> (52.6251, 62.15)
  line L775 (52.6251, 62.15) -> (66.6244, 62.15)
  line L776 (66.6244, 62.15) -> (66.6244, 63.1491)
  line L777 (66.6244, 63.1491) -> (67.4252, 63.1491)
  line L778 (67.4252, 63.1491) -> (67.4252, 66.2496)
  line L779 (67.4252, 66.2496) -> (66.6244, 66.2496)
  line L780 (66.6244, 66.2496) -> (66.6244, 72.0497)
  line L781 (66.6244, 72.0497) -> (67.4252, 72.0497)
  line L782 (67.4252, 72.0497) -> (67.4252, 75.1492)
  line L783 (67.4252, 75.1492) -> (66.6244, 75.1492)
  line L784 (66.6244, 75.1492) -> (66.6244, 76.1493)
  line L785 (66.6244, 76.1493) -> (52.6251, 76.1493)
  line L786 (71.6751, 76.1493) -> (71.6751, 75.1492)
  line L787 (71.6751, 75.1492) -> (70.8757, 75.1492)
  line L788 (70.8757, 75.1492) -> (70.8757, 72.0497)
  line L789 (70.8757, 72.0497) -> (71.6751, 72.0497)
  line L790 (71.6751, 72.0497) -> (71.6751, 66.2496)
  line L791 (71.6751, 66.2496) -> (70.8757, 66.2496)
  line L792 (70.8757, 66.2496) -> (70.8757, 63.1491)
  line L793 (70.8757, 63.1491) -> (71.6751, 63.1491)
  line L794 (71.6751, 63.1491) -> (71.6751, 62.15)
  line L795 (71.6751, 62.15) -> (85.6744, 62.15)
  line L796 (85.6744, 62.15) -> (85.6744, 63.1491)
  line L797 (85.6744, 63.1491) -> (86.4752, 63.1491)
  line L798 (86.4752, 63.1491) -> (86.4752, 66.2496)
  line L799 (86.4752, 66.2496) -> (85.6744, 66.2496)
  line L800 (85.6744, 66.2496) -> (85.6744, 72.0497)
  line L801 (85.6744, 72.0497) -> (86.4752, 72.0497)
  line L802 (86.4752, 72.0497) -> (86.4752, 75.1492)
  line L803 (86.4752, 75.1492) -> (85.6744, 75.1492)
  line L804 (85.6744, 75.1492) -> (85.6744, 76.1493)
  line L805 (85.6744, 76.1493) -> (71.6751, 76.1493)
  line L806 (90.7251, 76.1493) -> (90.7251, 75.1492)
  line L807 (90.7251, 75.1492) -> (89.9257, 75.1492)
  line L808 (89.9257, 75.1492) -> (89.9257, 72.0497)
  line L809 (89.9257, 72.0497) -> (90.7251, 72.0497)
  line L810 (90.7251, 72.0497) -> (90.7251, 66.2496)
  line L811 (90.7251, 66.2496) -> (89.9257, 66.2496)
  line L812 (89.9257, 66.2496) -> (89.9257, 63.1491)
  line L813 (89.9257, 63.1491) -> (90.7251, 63.1491)
  line L814 (90.7251, 63.1491) -> (90.7251, 62.15)
  line L815 (90.7251, 62.15) -> (104.7244, 62.15)
  line L816 (104.7244, 62.15) -> (104.7244, 63.1491)
  line L817 (104.7244, 63.1491) -> (105.5254, 63.1491)
  line L818 (105.5254, 63.1491) -> (105.5254, 66.2496)
  line L819 (105.5254, 66.2496) -> (104.7244, 66.2496)
  line L820 (104.7244, 66.2496) -> (104.7244, 72.0497)
  line L821 (104.7244, 72.0497) -> (105.5254, 72.0497)
  line L822 (105.5254, 72.0497) -> (105.5254, 75.1492)
  line L823 (105.5254, 75.1492) -> (104.7244, 75.1492)
  line L824 (104.7244, 75.1492) -> (104.7244, 76.1493)
  line L825 (104.7244, 76.1493) -> (90.7251, 76.1493)
  line L826 (109.7754, 76.1493) -> (109.7754, 75.1492)
  line L827 (109.7754, 75.1492) -> (108.9754, 75.1492)
  line L828 (108.9754, 75.1492) -> (108.9754, 72.0497)
  line L829 (108.9754, 72.0497) -> (109.7754, 72.0497)
  line L830 (109.7754, 72.0497) -> (109.7754, 66.2496)
  line L831 (109.7754, 66.2496) -> (108.9754, 66.2496)
  line L832 (108.9754, 66.2496) -> (108.9754, 63.1491)
  line L833 (108.9754, 63.1491) -> (109.7754, 63.1491)
  line L834 (109.7754, 63.1491) -> (109.7754, 62.15)
  line L835 (109.7754, 62.15) -> (123.7744, 62.15)
  line L836 (123.7744, 62.15) -> (123.7744, 63.1491)
  line L837 (123.7744, 63.1491) -> (124.5754, 63.1491)
  line L838 (124.5754, 63.1491) -> (124.5754, 66.2496)
  line L839 (124.5754, 66.2496) -> (123.7744, 66.2496)
  line L840 (123.7744, 66.2496) -> (123.7744, 72.0497)
  line L841 (123.7744, 72.0497) -> (124.5754, 72.0497)
  line L842 (124.5754, 72.0497) -> (124.5754, 75.1492)
  line L843 (124.5754, 75.1492) -> (123.7744, 75.1492)
  line L844 (123.7744, 75.1492) -> (123.7744, 76.1493)
  line L845 (123.7744, 76.1493) -> (109.7754, 76.1493)
  line L846 (128.8254, 76.1493) -> (128.8254, 75.1492)
  line L847 (128.8254, 75.1492) -> (128.0244, 75.1492)
  line L848 (128.0244, 75.1492) -> (128.0244, 72.0497)
  line L849 (128.0244, 72.0497) -> (128.8254, 72.0497)
  line L850 (128.8254, 72.0497) -> (128.8254, 66.2496)
  line L851 (128.8254, 66.2496) -> (128.0244, 66.2496)
  line L852 (128.0244, 66.2496) -> (128.0244, 63.1491)
  line L853 (128.0244, 63.1491) -> (128.8254, 63.1491)
  line L854 (128.8254, 63.1491) -> (128.8254, 62.15)
  line L855 (128.8254, 62.15) -> (142.8244, 62.15)
  line L856 (142.8244, 62.15) -> (142.8244, 63.1491)
  line L857 (142.8244, 63.1491) -> (143.6254, 63.1491)
  line L858 (143.6254, 63.1491) -> (143.6254, 66.2496)
  line L859 (143.6254, 66.2496) -> (142.8244, 66.2496)
  line L860 (142.8244, 66.2496) -> (142.8244, 72.0497)
  line L861 (142.8244, 72.0497) -> (143.6254, 72.0497)
  line L862 (143.6254, 72.0497) -> (143.6254, 75.1492)
  line L863 (143.6254, 75.1492) -> (142.8244, 75.1492)
  line L864 (142.8244, 75.1492) -> (142.8244, 76.1493)
  line L865 (142.8244, 76.1493) -> (128.8254, 76.1493)
  line L866 (147.8754, 76.1493) -> (147.8754, 75.1492)
  line L867 (147.8754, 75.1492) -> (147.0754, 75.1492)
  line L868 (147.0754, 75.1492) -> (147.0754, 72.0497)
  line L869 (147.0754, 72.0497) -> (147.8754, 72.0497)
  line L870 (147.8754, 72.0497) -> (147.8754, 66.2496)
  line L871 (147.8754, 66.2496) -> (147.0754, 66.2496)
  line L872 (147.0754, 66.2496) -> (147.0754, 63.1491)
  line L873 (147.0754, 63.1491) -> (147.8754, 63.1491)
  line L874 (147.8754, 63.1491) -> (147.8754, 62.15)
  line L875 (147.8754, 62.15) -> (161.8744, 62.15)
  line L876 (161.8744, 62.15) -> (161.8744, 63.1491)
  line L877 (161.8744, 63.1491) -> (162.6754, 63.1491)
  line L878 (162.6754, 63.1491) -> (162.6754, 66.2496)
  line L879 (162.6754, 66.2496) -> (161.8744, 66.2496)
  line L880 (161.8744, 66.2496) -> (161.8744, 72.0497)
  line L881 (161.8744, 72.0497) -> (162.6754, 72.0497)
  line L882 (162.6754, 72.0497) -> (162.6754, 75.1492)
  line L883 (162.6754, 75.1492) -> (161.8744, 75.1492)
  line L884 (161.8744, 75.1492) -> (161.8744, 76.1493)
  line L885 (161.8744, 76.1493) -> (147.8754, 76.1493)
  line L886 (166.9254, 76.1493) -> (166.9254, 75.1492)
  line L887 (166.9254, 75.1492) -> (166.1254, 75.1492)
  line L888 (166.1254, 75.1492) -> (166.1254, 72.0497)
  line L889 (166.1254, 72.0497) -> (166.9254, 72.0497)
  line L890 (166.9254, 72.0497) -> (166.9254, 66.2496)
  line L891 (166.9254, 66.2496) -> (166.1254, 66.2496)
  line L892 (166.1254, 66.2496) -> (166.1254, 63.1491)
  line L893 (166.1254, 63.1491) -> (166.9254, 63.1491)
  line L894 (166.9254, 63.1491) -> (166.9254, 62.15)
  line L895 (166.9254, 62.15) -> (180.9244, 62.15)
  line L896 (180.9244, 62.15) -> (180.9244, 63.1491)
  line L897 (180.9244, 63.1491) -> (181.7254, 63.1491)
  line L898 (181.7254, 63.1491) -> (181.7254, 66.2496)
  line L899 (181.7254, 66.2496) -> (180.9244, 66.2496)
  line L900 (180.9244, 66.2496) -> (180.9244, 72.0497)
  line L901 (180.9244, 72.0497) -> (181.7254, 72.0497)
  line L902 (181.7254, 72.0497) -> (181.7254, 75.1492)
  line L903 (181.7254, 75.1492) -> (180.9244, 75.1492)
  line L904 (180.9244, 75.1492) -> (180.9244, 76.1493)
  line L905 (180.9244, 76.1493) -> (166.9254, 76.1493)
  line L906 (185.9754, 76.1493) -> (185.9754, 75.1492)
  line L907 (185.9754, 75.1492) -> (185.1754, 75.1492)
  line L908 (185.1754, 75.1492) -> (185.1754, 72.0497)
  line L909 (185.1754, 72.0497) -> (185.9754, 72.0497)
  line L910 (185.9754, 72.0497) -> (185.9754, 66.2496)
  line L911 (185.9754, 66.2496) -> (185.1754, 66.2496)
  line L912 (185.1754, 66.2496) -> (185.1754, 63.1491)
  line L913 (185.1754, 63.1491) -> (185.9754, 63.1491)
  line L914 (185.9754, 63.1491) -> (185.9754, 62.15)
  line L915 (185.9754, 62.15) -> (199.9744, 62.15)
  line L916 (199.9744, 62.15) -> (199.9744, 63.1491)
  line L917 (199.9744, 63.1491) -> (200.7754, 63.1491)
  line L918 (200.7754, 63.1491) -> (200.7754, 66.2496)
  line L919 (200.7754, 66.2496) -> (199.9744, 66.2496)
  line L920 (199.9744, 66.2496) -> (199.9744, 72.0497)
  line L921 (199.9744, 72.0497) -> (200.7754, 72.0497)
  line L922 (200.7754, 72.0497) -> (200.7754, 75.1492)
  line L923 (200.7754, 75.1492) -> (199.9744, 75.1492)
  line L924 (199.9744, 75.1492) -> (199.9744, 76.1493)
  line L925 (199.9744, 76.1493) -> (185.9754, 76.1493)
  line L926 (205.0254, 76.1493) -> (205.0254, 75.1492)